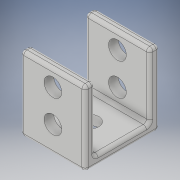
# Autodesk Inventor part: top printhead screwplate2
Saved by Autodesk Inventor 2019 (Build 230136000, 136)
## iProperties
Created: 2018-10-02
Part Number: top printhead screwplate2
Material: Generic
Document SubType Name: Modeling
Designer: Iek Man Lei
Density: 1 g/cm^3
Appearance: Default
Author: Iek Man Lei
Autodesk Inventor part; units mm, degrees
ref_plane "YZ Plane" through (0, 0, 0) normal (1, 0, 0) x (0, 1, 0)
ref_plane "XZ Plane" through (0, 0, 0) normal (0, 1, 0) x (-1, 0, 0)
ref_plane "XY Plane" through (0, 0, 0) normal (0, 0, 1) x (1, 0, 0)
sketch "Sketch1" plane through (0, 0, 0) normal (0, 1, 0) x (-1, 0, 0)
  line L0 (14.2, 15.6875) -> (-5.8, 15.6875)
  line L1 (-5.8, 15.6875) -> (-5.8, -7.3125)
  line L2 (-5.8, -7.3125) -> (14.2, -7.3125)
  line L3 (14.2, -7.3125) -> (14.2, 15.6875)
  circle A0 centre (4.2, 4.1875) radius 2.75
  point P0 (0, 0)
  dimension "d0" = 20
  dimension "d1" = 23
  dimension "d9" = 5.5
  dimension "d10" = 11.5
  dimension "d11" = 10
  constraints: 8 end point, 2 parallel, 1 centre point, 1 horizontal, 1 perpendicular
  measures "d0" distance of L0.start L0.end
  measures "d1" distance of L0.end L1.end
  measures "d9" diameter of A0
  measures "d10" distance from line of L2 A0.centre
  measures "d11" distance from line of L3 A0.centre
extrude "Extrusion2" add sketch "Sketch1" along normal blind 3
sketch "Sketch3" plane through (0, 3, 0) normal (0, 1, 0) x (1, 0, 0)
  line L0 (5.8, -15.6875) -> (5.8, 7.3125) projected
  line L1 (-14.2, -15.6875) -> (5.8, -15.6875) projected
  line L2 (5.8, -12.6875) -> (-14.2, -12.6875)
  line L3 (-14.2, -12.6875) -> (-14.2, -15.6875)
  line L4 (-14.2, -15.6875) -> (5.8, -15.6875)
  line L5 (5.8, -15.6875) -> (5.8, -12.6875)
  line L6 (5.8, 7.3125) -> (-14.2, 7.3125) projected
  line L7 (5.8, 4.3125) -> (-14.2, 4.3125)
  line L8 (-14.2, 4.3125) -> (-14.2, 7.3125)
  line L9 (-14.2, 7.3125) -> (5.8, 7.3125)
  line L10 (5.8, 7.3125) -> (5.8, 4.3125)
  point P0 (0, 0)
  dimension "d14" = 3
  dimension "d15" = 3
  constraints: 16 end point, 4 parallel, 2 horizontal, 2 perpendicular, 2 point on line
  measures "d14" distance of L2.end L1.start
  measures "d15" distance of L7.end L6.end
extrude "Extrusion3" add sketch "Sketch3" along normal blind 20
sketch "Sketch4" plane through (-14.2, 0, 15.6875) normal (0, 0, 1) x (1, 0, 0)
  circle A0 centre (10, 8) radius 2.75
  circle A1 centre (10, 18) radius 2.75
  line L0 (0, 0) -> (20, 0) projected
  line L1 (0, 23) -> (20, 23) projected
  line L2 (20, 0) -> (20, 23) projected
  line L3 (0, 3) -> (20, 3) projected
  point P0 (14.2, 0)
  dimension "d18" = 5.5
  dimension "d19" = 5.5
  dimension "d21" = 5
  dimension "d22" = 10
  dimension "d25" = 5
  constraints: 2 centre point, 1 vertical alignment
  measures "d18" diameter of A0
  measures "d19" diameter of A1
  measures "d21" distance from line of L1 A1.centre
  measures "d22" distance from line of L2 A0.centre
  measures "d25" distance from line of L3 A0.centre
extrude "Extrusion4" cut sketch "Sketch4" against normal through all
fillet "Fillet1" radius 1 24 edges at (-14.2, 3, 4.1875) (-14.2, 13, -4.3125) (5.8, 3, 4.1875) (-14.2, 0, 4.1875) (-14.2, 11.5, -7.3125) (-14.2, 23, -5.8125) (5.8, 23, -5.8125) (-14.2, 23, 14.1875) (-4.2, 23, 12.6875) (-14.2, 13, 12.6875) (-4.2, 23, -4.3125) (-4.2, 23, -7.3125) (5.8, 13, -4.3125) (5.8, 11.5, -7.3125) (5.8, 0, 4.1875) (5.8, 11.5, 15.6875) (5.8, 13, 12.6875) (-4.2, 23, 15.6875) (5.8, 23, 14.1875) (-14.2, 11.5, 15.6875) (-4.2, 0, 15.6875) (-4.2, 0, -7.3125) (-4.2, 3, 12.6875) (-4.2, 3, -4.3125)
body "Solid2"
